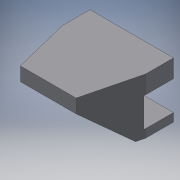
# Autodesk Inventor part: ma_3d1
Saved by Autodesk Inventor 2018.2 (Build 222227000, 227)
## iProperties
Created: 2018-05-15
Part Number: ma_3d1
Material: 一般
Document SubType Name: Modeling
Designer: SHUICHI
Density: 1 g/cm^3
Appearance: 既定
Author: SHUICHI
Autodesk Inventor part; units mm, degrees
ref_plane "YZ Plane" through (0, 0, 0) normal (1, 0, 0) x (0, 1, 0)
ref_plane "XZ Plane" through (0, 0, 0) normal (0, 1, 0) x (-1, 0, 0)
ref_plane "XY Plane" through (0, 0, 0) normal (0, 0, 1) x (1, 0, 0)
sketch "スケッチ1" plane through (0, 0, 0) normal (0, 0, 1) x (1, 0, 0)
  line L0 (0, 0) -> (0, -12)
  line L1 (0, -12) -> (-2, -40)
  line L2 (-2, -40) -> (-28, -40)
  line L3 (-28, -40) -> (-30, -12)
  line L4 (-30, -12) -> (-30, 0)
  line L5 (-30, 0) -> (0, 0)
  circle A0 centre (-25, -5) radius 1.75
  circle A1 centre (-5, -5) radius 1.75
  dimension "d0" = 12
  dimension "d1" = 30
  dimension "d2" = 40
  dimension "d3" = 2
  dimension "d4" = 26
  dimension "d12" = 3.5
  dimension "d13" = 3.5
  dimension "d14" = 5
  dimension "d15" = 5
  dimension "d16" = 5
  constraints: 12 end point, 2 centre point, 2 horizontal alignment, 1 parallel, 1 perpendicular, 1 vertical
  measures "d0" distance of L0.start L0.end
  measures "d1" distance of L4.end L0.start
  measures "d2" distance between parallel lines of L5 L2
  measures "d3" horizontal distance of L0.end L1.end
  measures "d4" distance of L1.end L2.end
  measures "d12" diameter of A0
  measures "d13" diameter of A1
  measures "d14" distance from line of L4 A0.centre
  measures "d15" distance from line of L0 A1.centre
  measures "d16" distance from line of L5 A0.centre
extrude "押し出し1" add sketch "スケッチ1" along normal blind 20
sketch "スケッチ2" plane through (0, -12, 0) normal (1, 0, 0) x (0, 0, -1)
  line L0 (0, 12) -> (-20, 12) projected
  line L1 (-3, 12) -> (-13.5, 12)
  line L2 (-13.5, 12) -> (-13.5, 1.5)
  line L3 (-13.5, 1.5) -> (-3, 1.5)
  line L4 (-3, 1.5) -> (-3, 12)
  line L5 (0, 12) -> (0, 0) projected
  line L6 (0, -28) -> (0, 0) projected
  line L7 (0, 0) -> (-12, -28)
  line L8 (0, -28) -> (-20, -28) projected
  circle A0 centre (-16, -23) radius 1.75
  line L9 (-20, -28) -> (-20, 0) projected
  dimension "d7" = 10.5
  dimension "d8" = 10.5
  dimension "d9" = 3
  dimension "d22" = 12
  dimension "d34" = 3.5
  dimension "d35" = 4
  dimension "d36" = 5
  constraints: 10 end point, 2 parallel, 2 point on line, 1 centre point, 1 horizontal, 1 perpendicular
  measures "d7" distance of L3.end L2.end
  measures "d8" distance of L2.end L1.end
  measures "d9" distance between parallel lines of L5 L4
  measures "d22" horizontal distance of L5.end L7.end
  measures "d34" diameter of A0
  measures "d35" distance from line of L9 A0.centre
  measures "d36" distance from line of L8 A0.centre
extrude "押し出し2" cut sketch "スケッチ2" against normal through all
sketch "スケッチ3" plane through (0, 0, 0) normal (0, 0, -1) x (-1, 0, 0)
  line L0 (4, -40) -> (26, -40)
  line L1 (26, -40) -> (26, -16.5)
  line L2 (26, -16.5) -> (4, -16.5)
  line L3 (4, -16.5) -> (4, -40)
  line L4 (28, -40) -> (2, -40) projected
  point P0 (0, 0)
  dimension "d17" = 23.5
  dimension "d18" = 2
  dimension "d19" = 2
  constraints: 8 end point, 2 parallel, 1 collinear, 1 horizontal, 1 perpendicular
  measures "d17" distance of L2.end L0.start
  measures "d18" distance from line of L4.end L3
  measures "d19" distance from line of L4.start L1
extrude "押し出し3" cut sketch "スケッチ3" against normal blind 12
sketch "スケッチ4" plane through (0, 0, 20) normal (0, 0, 1) x (1, 0, 0)
  line L0 (-22.5, -30) -> (-7.5, -30)
  line L1 (-7.5, -30) -> (-7.5, -20)
  line L2 (-7.5, -20) -> (-22.5, -20)
  line L3 (-22.5, -20) -> (-22.5, -30)
  line L4 (0, 0) -> (-30, 0) projected
  line L5 (0, -12) -> (0, 0) projected
  dimension "d23" = 15
  dimension "d24" = 20
  dimension "d25" = 7.5
  dimension "d26" = 10
  constraints: 8 end point, 4 coincident, 2 parallel, 1 horizontal, 1 perpendicular
  measures "d23" distance of L2.end L1.end
  measures "d24" distance between parallel lines of L4 L2
  measures "d25" distance between parallel lines of L5 L1
  measures "d26" distance of L0.end L1.end
hole "穴1" at (-22.5, -20, 20) at (-22.5, -30, 20) at (-7.5, -30, 20) at (-7.5, -20, 20) direction (0, 0, -1) diameter 3.2 end through all
fillet "フィレット1" radius 2 7 edges at (-26, -16.5, 6.9643) (-4, -16.5, 6.9643) (-15, -40, 12) (-3, -40, 12) (-27, -40, 12) (0, -12, 10) (-30, -12, 10)
fillet "フィレット2" radius 2 4 edges at (0, 0, 16.75) (0, 0, 1.5) (-30, 0, 1.5) (-30, 0, 16.75)
